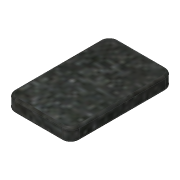
# Autodesk Inventor part: 6AESC
Saved by Autodesk Inventor 2019 (Build 230136000, 136)
## iProperties
Created: 2022-04-09
Part Number: 6AESC
Material: Steel
Document SubType Name: Modeling
Designer: solyo
Density: 7.85 g/cm^3
Appearance: Plate
Mass: 8.33492 g
Surface Area: 9.04605 cm^2
Volume: 1.06177 cm^3
Author: solyo
Autodesk Inventor part; units mm, degrees
ref_plane "YZ Plane" through (0, 0, 0) normal (1, 0, 0) x (0, 1, 0)
ref_plane "XZ Plane" through (0, 0, 0) normal (0, 1, 0) x (-1, 0, 0)
ref_plane "XY Plane" through (0, 0, 0) normal (0, 0, 1) x (1, 0, 0)
sketch "Sketch1" plane through (0, 0, 0) normal (0, 0, 1) x (1, 0, 0)
  line L0 (7.5, -1.5) -> (-7.5, -1.5)
  line L1 (-7.5, -1.5) -> (-7.5, 1.5)
  line L2 (-7.5, 1.5) -> (7.5, 1.5)
  line L3 (7.5, 1.5) -> (7.5, -1.5)
  line L4 (7.5, -1.5) -> (-7.5, 1.5) construction
  line L5 (-7.5, -1.5) -> (7.5, 1.5) construction
  point P0 (0, 0)
  dimension "d0" = 15
  dimension "d1" = 3
  constraints: 12 end point, 2 midpoint, 2 parallel, 1 horizontal, 1 perpendicular
  measures "d0" distance of L1.end L2.end
  measures "d1" distance of L0.end L1.end
extrude "Extrusion1" add sketch "Sketch1" along normal mid plane 24
fillet "Fillet1" radius 2 4 edges at (7.5, 0, 12) (-7.5, 0, 12) (-7.5, 0, -12) (7.5, 0, -12)
fillet "Fillet1" radius 0.5 8 edges at (-7.5, 1.5, 0) (0, 1.5, -12) (7.5, 1.5, 0) (0, 1.5, 12) (0, -1.5, 12) (7.5, -1.5, 0) (0, -1.5, -12) (-7.5, -1.5, 0)
body "Solid1"
